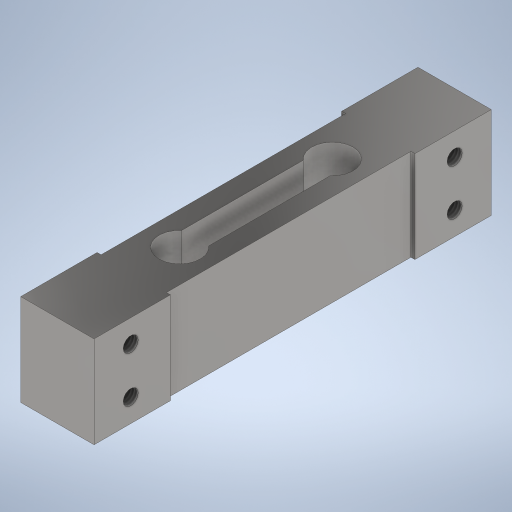
# Autodesk Inventor part: Célula de carga
Saved by Autodesk Inventor 2023 (Build 270158000, 158)
## iProperties
Created: 2023-03-25
Part Number: Célula de carga
Material: Aço inoxidável
Document SubType Name: Sheet Metal
Designer: Mateus
Density: 8 g/cm^3
Sheet Metal Rule: Default_mm
Appearance: Aço - Polido
Mass: 518.867 g
Surface Area: 186.075 cm^2
Volume: 64.8584 cm^3
Author: Mateus
Autodesk Inventor part; units mm, degrees
ref_plane "YZ Plane" through (0, 0, 0) normal (1, 0, 0) x (0, 1, 0)
ref_plane "XZ Plane" through (0, 0, 0) normal (0, 1, 0) x (-1, 0, 0)
ref_plane "XY Plane" through (0, 0, 0) normal (0, 0, 1) x (1, 0, 0)
sketch "Esboço1" plane through (0, 0, 0) normal (0, 1, 0) x (-1, 0, 0)
  line L0 (0, 0) -> (24, 0)
  line L1 (24, -130) -> (0, -130)
  arc A0 (16.4, -45.1188) -> (7.6, -45.1188) centre (12, -40) ccw
  arc A1 (7.6, -84.8812) -> (16.4, -84.8812) centre (12, -90) ccw
  line L2 (7.6, -45.1188) -> (7.6, -84.8812)
  line L3 (16.4, -84.8812) -> (16.4, -45.1188)
  line L4 (24, -25) -> (22.7, -25)
  line L5 (22.7, -25) -> (22.7, -105)
  line L6 (22.7, -105) -> (24, -105)
  line L7 (1.3, -25) -> (0, -25)
  line L8 (0, -105) -> (1.3, -105)
  line L9 (1.3, -105) -> (1.3, -25)
  line L10 (24, 0) -> (24, -25)
  line L11 (24, -105) -> (24, -130)
  line L12 (0, -130) -> (0, -105)
  line L13 (0, -25) -> (0, 0)
  line L14 (7.6, -65) -> (1.3, -65)
  line L15 (1.3, -65) -> (22.7, -65)
  line L16 (12, -65) -> (12, -130)
  line L17 (12, -90) -> (12, -130)
  point P0 (12, 0)
  point P1 (12, -55.1552)
  point P2 (-50.7156, -65)
  dimension "d0" = 24
  dimension "d1" = 130
  dimension "d2" = 13.5
  dimension "d8" = 0
  dimension "d9" = 1.3
  dimension "d10" = 80
  dimension "d11" = 1.3
  dimension "d12" = 80
  dimension "d15" = 0
  dimension "d16" = 0
  dimension "d34" = 8.8
  dimension "d37" = 0
  dimension "d38" = 4.4
  dimension "d39" = 50
  dimension "d40" = 25
  dimension "d41" = 25
  constraints: 36 end point, 8 parallel, 5 horizontal, 5 midpoint, 4 perpendicular, 4 point on circle, 3 vertical, 2 centre point, 2 collinear, 1 equal radius
  measures "d0" distance of L1.start L1.end
  measures "d1" distance of L0.end L1.start
  measures "d2" diameter of A0
  measures "d8" horizontal distance of L17.start point (12, -55.155)
  measures "d9" distance of L6.end L5.end
  measures "d10" distance of L5.end L4.end
  measures "d11" distance of L8.end L8.start
  measures "d12" distance of L8.start L7.end
  measures "d15" distance of point (22.7, -65) L15.end
  measures "d16" vertical distance of point (-50.716, -65) L14.end
  measures "d34" distance from line of L14.start L3
  measures "d37" horizontal distance of L17.start A0.centre
  measures "d38" horizontal distance of point (12, -55.155) L14.start
  measures "d39" distance of A0.centre L17.start
  measures "d40" distance of L6.end L1.start
  measures "d41" distance of L1.end L8.start
extrude "Extrusão1" add sketch "Esboço1" along normal blind 30 contours L0 L10 L4 L5 L15 L3 A0 L2 L14 L9 L7 L13 | L14 L2 A1 L16 L1 L12 L8 L9 | L5 L6 L11 L1 L16 A1 L3 L15
sketch "Esboço2" plane through (0, 0, 0) normal (1, 0, 0) x (0, 0, -1)
  line L0 (0, 0) -> (0, 30) projected
  line L1 (130, 0) -> (130, 30) projected
  line L2 (0, 30) -> (25, 30) projected
  line L3 (0, 0) -> (25, 0) projected
  line L4 (105, 30) -> (130, 30) projected
  line L5 (105, 0) -> (130, 0) projected
  point P0 (12, 22.5)
  point P1 (12, 7.5)
  point P2 (118, 22.5)
  point P3 (118, 7.5)
  point P4 (117.5, 0)
  dimension "d19" = 12
  dimension "d20" = 12
  dimension "d21" = 12
  dimension "d22" = 12
  dimension "d23" = 7.5
  dimension "d24" = 7.5
  dimension "d25" = 7.5
  dimension "d26" = 7.5
  constraints: 1 midpoint
  measures "d19" distance from line of L0 point (12, 22.5)
  measures "d20" distance from line of L0 point (12, 7.5)
  measures "d21" distance from line of L1 point (118, 22.5)
  measures "d22" distance from line of L1 point (118, 7.5)
  measures "d23" distance from line of L2 point (12, 22.5)
  measures "d24" distance from line of L3 point (12, 7.5)
  measures "d25" distance from line of L4 point (118, 22.5)
  measures "d26" vertical distance of point (117.5, 0) point (118, 7.5)
hole "Furo1" at (0, 22.5, -12) at (0, 7.5, -12) at (0, 22.5, -118) at (0, 7.5, -118) direction (-1, 0, 0) diameter 4.917 end through all thread size "M6x1" class "6H" standard "ISO Metric profile"
equation "\"d38\" = 0.5 * d34"
equation "\"d20\" = d19"
equation "\"d21\" = d19"
equation "\"d22\" = d19"
equation "\"d24\" = d23"
equation "\"d25\" = d23"
equation "\"d26\" = d24"
equation "\"Raio_vergadura\" = Espessura"
equation "\"Largura_alívio_de_vergadura\" = Espessura"
equation "\"Profundidade_alívio_de_vergadura\" = 0.5 * Espessura"
equation "\"Tamanho_alívio_de_dobra\" = 4 * Espessura"
equation "\"Remanescente_mínimo\" = 2 * Espessura"
equation "\"Raiodetransição\" = Raio_vergadura"
equation "\"Tamanho_de_raio_de_Jacobi\" = Raio_vergadura"
equation "\"TamanhoFolga\" = Espessura"
equation "\"d3\" = 0.5 * d0"
equation "\"d4\" = 0.5 * d0"
equation "\"Espessura\" = 0.5"
